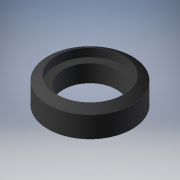
# Autodesk Inventor part: 20_Beamexpander_Lens_Adapter
Saved by Autodesk Inventor 2019 (Build 230136000, 136)
## iProperties
Created: 2019-04-26
Part Number: 20_Beamexpander_Lens_Adapter
Material: Generic
Document SubType Name: Modeling
Designer: diederichbenedict
Density: 1 g/cm^3
Appearance: Default
Author: diederichbenedict
Autodesk Inventor part; units mm, degrees
ref_plane "YZ Plane" through (0, 0, 0) normal (1, 0, 0) x (0, 1, 0)
ref_plane "XZ Plane" through (0, 0, 0) normal (0, 1, 0) x (-1, 0, 0)
ref_plane "XY Plane" through (0, 0, 0) normal (0, 0, 1) x (1, 0, 0)
sketch "Sketch1" plane through (0, 0, 0) normal (1, 0, 0) x (0, 1, 0)
  line L0 (0, 0) -> (0, -8)
  line L1 (0, 0) -> (8, 0) construction
  line L2 (0, -8) -> (4, -8)
  arc A0 (4, -8) -> (6.5, 0) centre (-9.2716, 0.538) ccw
  line L3 (6.5, 0) -> (0, 0)
  line L4 (4.9022, -6.4) -> (3.3022, -6.4)
  line L5 (3.3022, -6.4) -> (3.3022, 0)
  line L6 (0, 0) -> (3.3022, 0)
  line L7 (3.3022, -5.0708) -> (0, -5.0708)
  dimension "d0" = 8
  dimension "d1" = 90
  dimension "d2" = 4
  dimension "d3" = 90
  dimension "d4" = 6.5
  dimension "d6" = 6.4
  dimension "d7" = 1.6
  constraints: 16 end point, 4 perpendicular, 4 point on line, 3 horizontal, 3 point on circle, 1 centre point, 1 collinear, 1 vertical
  measures "d0" distance of L0.start L0.end
  measures "d1" angle of L0 L1
  measures "d2" distance of L0.end L2.end
  measures "d3" angle of L2 L0
  measures "d4" distance of L3.start L0.start
  measures "d6" distance between parallel lines of L1 L4
  measures "d7" distance of L4.start L4.end
revolve "Revolution1" add sketch "Sketch1" angle 360 about axis through (0, 6.5, 0) along (0, -1, 0) contours L7 L5 L4 A0 L2 L0
body "Solid1"
